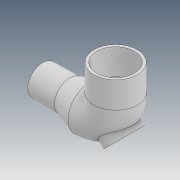
# Autodesk Inventor part: Ambu90deg
Saved by Autodesk Inventor 2020 (Build 240168000, 168)
## iProperties
Created: 2020-04-26
Part Number: Ambu90deg
Material: Generic
Document SubType Name: Modeling
Designer: Theo Cominotto
Density: 1 g/cm^3
Appearance: Default
Author: Theo Cominotto
Autodesk Inventor part; units mm, degrees
sketch "Sketch1" plane through (0, 0, 0) normal (0, 0, 1) x (1, 0, 0)
  line L0 (15, 28.2088) -> (15.15, 10.0588)
  line L1 (13, 28.2088) -> (13.15, 10.0588)
  line L2 (13.15, 10.0588) -> (13.1595, 8.9045)
  line L3 (15.15, 10.0588) -> (15.1653, 8.2088)
  line L4 (15.1653, 8.2088) -> (10.25, -5.7912)
  line L5 (10.25, -5.7912) -> (10.25, -5.7912)
  line L6 (8, -5.7712) -> (8, -5.7912)
  line L7 (13.1595, 8.9045) -> (8, -5.7912)
  line L8 (15, 28.2088) -> (13, 28.2088)
  line L9 (0, -12.5912) -> (0, 35.0088) construction
  line L10 (-1, 0) -> (-1, 28.2088) construction
  line L11 (10.25, -5.7912) -> (8, -5.7912)
  line L12 (13.1595, 8.9045) -> (15.1595, 8.9045)
  point P0 (0, 0)
  point P1 (0, 0)
  point P2 (-1, 22.6667)
  dimension "d0" = 2
  dimension "d1" = 2
  dimension "d2" = 0
  dimension "d3" = 0
  dimension "d4" = 18.15
  dimension "d5" = 1.9999
  dimension "d6" = 14
  dimension "d7" = 0
  dimension "d8" = 1.85
  dimension "d9" = 2.123
  dimension "d10" = 1
  constraints: 24 end point, 2 collinear, 2 horizontal, 2 vertical, 1 parallel, 1 point on line
  measures "d0" distance of L0.end L2.start
  measures "d1" distance of L1.start L0.start
  measures "d2" vertical distance of L0.end L2.start
  measures "d3" vertical distance of L0.start L1.start
  measures "d4" vertical distance of L0.start L0.end
  measures "d5" distance between parallel lines of L1 L0
  measures "d6" vertical distance of L3.end L4.end
  measures "d7" distance of L4.end L5.end
  measures "d8" vertical distance of L0.end L3.end
  measures "d9" distance between parallel lines of L7 L4
  measures "d10" distance between parallel lines of L9 L10
revolve "Revolution1" add sketch "Sketch1" angle 360 about axis through (-1, 0, 0) along (0, 1, 0) contours L0 L3 L12 L2 L1 L8
ref_plane "Work Plane1" through (-20, 0, 0) normal (1, 0, 0) x (0, 1, 0)
sketch "Sketch2" plane through (-20, 0, 0) normal (1, 0, 0) x (0, 1, 0)
  line L0 (8.9045, 14.1595) -> (8.9045, -14.1595) construction
  line L1 (8.9045, 0) -> (-10.0955, 0) construction
  point P0 (0, 0)
  dimension "d13" = 19
  constraints: 2 end point, 1 horizontal, 1 midpoint
  measures "d13" distance of L1.start L1.end
sketch "Sketch3" plane through (-1, 8.9045, 0) normal (0, -1, 0) x (1, 0, 0)
  circle A0 centre (0, 0) radius 16.1595 projected
  circle A1 centre (0, 0) radius 14.1595 projected
  point P0 (1, 0)
revolve "Revolution2" add sketch "Sketch3" angle 90 about axis through (-20, 8.9045, 14.1595) along (0, 0, -1)
ref_plane "Work Plane2" through (0, 0, 0) normal (0, 0, 1) x (1, 0, 0)
sketch "Sketch4" plane through (0, 0, 0) normal (0, 0, 1) x (1, 0, 0)
  line L0 (-20, 6.0641) -> (-20, -26.255) construction
  line L1 (-20, -10.0955) -> (-35, -10.0955) construction
  line L2 (-35, -10.0955) -> (-55, -10.0955) construction
  line L3 (-55, -10.0955) -> (-55, 0.9045) construction
  line L4 (-35, -10.0955) -> (-35, 1.1545) construction
  line L5 (-35, 1.1545) -> (-55, 0.9045)
  line L6 (-55, 0.9045) -> (-55, -0.2955)
  line L7 (-55, -0.2955) -> (-35, -0.0455)
  line L8 (-20, -24.255) -> (-20, 4.0641) projected
  line L9 (-20, 4.0641) -> (-35, -0.0455)
  line L10 (-35, 1.1545) -> (-20, 6.0641)
  line L11 (-20, 6.0641) -> (-20, 4.0641)
  point P0 (0, 0)
  dimension "d16" = 15
  dimension "d17" = 20
  dimension "d18" = 11
  dimension "d19" = 11.25
  dimension "d20" = 1.2
  dimension "d21" = 1.2
  constraints: 20 end point, 3 point on line, 2 vertical, 1 collinear, 1 horizontal, 1 midpoint
  measures "d16" distance of L1.start L1.end
  measures "d17" distance of L1.end L2.end
  measures "d18" distance of L2.end L3.end
  measures "d19" distance of L1.end L4.end
  measures "d20" distance of L3.end L6.end
  measures "d21" distance of L4.end L7.end
revolve "Revolution3" add sketch "Sketch4" angle 360 about axis through (-35, -10.0955, 0) along (-1, 0, 0)
ref_plane "Work Plane4" through (5.4558, -16.5513, 14.1595) normal (0.7071068, -0.7071068, 0) x (0, 0, -1)
ref_plane "Work Plane3" through (-20, 8.9045, 14.1595) normal (0.7071068, -0.7071068, 0) x (0, 0, -1)
sketch "Sketch5" plane through (5.4558, -16.5513, 14.1595) normal (0.7071068, -0.7071068, 0) x (0, 0, -1)
  circle A0 centre (14.1595, 0.0528) radius 12.5
  point P0 (14.1595, 7.8457)
  dimension "d25" = 25
  constraints: 1 centre point
  measures "d25" diameter of A0
extrude "Extrusion1" add sketch "Sketch5" against normal up to surface
body "Solid1"
